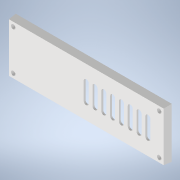
# Autodesk Inventor part: A-04
Saved by Autodesk Inventor 2022.2 (Build 262287000, 287)
## iProperties
Created: 2021-11-25
Part Number: A-04
Material: Generic
Document SubType Name: Modeling
Designer: kfcs7
Density: 1 g/cm^3
Appearance: Default
Author: kfcs7
Autodesk Inventor part; units mm, degrees
ref_plane "YZ Plane" through (0, 0, 0) normal (1, 0, 0) x (0, 1, 0)
ref_plane "XZ Plane" through (0, 0, 0) normal (0, 1, 0) x (-1, 0, 0)
ref_plane "XY Plane" through (0, 0, 0) normal (0, 0, 1) x (1, 0, 0)
sketch "Sketch1" plane through (0, 0, 0) normal (0, 0, 1) x (1, 0, 0)
  circle A0 centre (4, 4) radius 2.25 construction
  line L0 (119, 20) -> (119, 10.0711) construction
  line L1 (119, 10.0711) -> (113.9289, 5) construction
  line L2 (113.9289, 5) -> (10.0711, 5) construction
  line L3 (10.0711, 5) -> (5, 10.0711) construction
  line L4 (5, 10.0711) -> (5, 20) construction
  line L5 (0, 20) -> (5, 20) construction
  line L6 (0, 0) -> (0, 20) construction
  line L7 (124, 0) -> (0, 0) construction
  line L8 (124, 0) -> (124, 20) construction
  line L9 (119, 20) -> (124, 20) construction
  circle A1 centre (120, 4) radius 2.25 construction
  circle A2 centre (120, 36) radius 2.25 construction
  line L10 (119, 29.9289) -> (119, 20) construction
  line L11 (124, 20) -> (119, 20) construction
  line L12 (124, 40) -> (124, 20) construction
  line L13 (0, 40) -> (124, 40) construction
  line L14 (0, 20) -> (0, 40) construction
  line L15 (5, 20) -> (0, 20) construction
  line L16 (5, 20) -> (5, 29.9289) construction
  line L17 (5, 29.9289) -> (10.0711, 35) construction
  line L18 (10.0711, 35) -> (113.9289, 35) construction
  line L19 (113.9289, 35) -> (119, 29.9289) construction
  circle A3 centre (4, 36) radius 2.25 construction
  line L20 (124, 0) -> (0, 0)
  line L21 (0, 0) -> (0, 40)
  line L22 (0, 40) -> (124, 40)
  line L23 (124, 40) -> (124, 0)
  constraints: 8 end point, 2 parallel, 1 horizontal, 1 perpendicular
extrude "Extrusion1" add sketch "Sketch1" along normal blind 6 draft -5
sketch "Sketch4" plane through (0, 0, 0) normal (0, 0, -1) x (-1, 0, 0)
  line L0 (-124, 40) -> (0, 40) construction
  line L1 (-124, 0) -> (-124, 40) construction
  line L2 (0, 0) -> (-124, 0) construction
  line L3 (0, 40) -> (0, 0) construction
  circle A0 centre (-120, 4) radius 2.25 construction
  line L4 (-119, 10.0711) -> (-119, 20) projected
  line L5 (-124, 20) -> (-119, 20) construction
  line L6 (-124, 0) -> (-124, 20) construction
  line L7 (0, 0) -> (-124, 0) construction
  line L8 (0, 20) -> (0, 0) construction
  line L9 (-5, 20) -> (0, 20) construction
  line L10 (-5, 20) -> (-5, 10.0711) projected
  line L11 (-5, 10.0711) -> (-10.0711, 5) projected
  line L12 (-10.0711, 5) -> (-113.9289, 5) projected
  line L13 (-113.9289, 5) -> (-119, 10.0711) projected
  circle A1 centre (-4, 4) radius 2.25 construction
  circle A2 centre (-4, 36) radius 2.25 construction
  line L14 (-119, 20) -> (-119, 29.9289) projected
  line L15 (-119, 29.9289) -> (-113.9289, 35) projected
  line L16 (-113.9289, 35) -> (-10.0711, 35) projected
  line L17 (-10.0711, 35) -> (-5, 29.9289) projected
  line L18 (-5, 29.9289) -> (-5, 20) projected
  line L19 (0, 20) -> (-5, 20) construction
  line L20 (0, 40) -> (0, 20) construction
  line L21 (-124, 40) -> (0, 40) construction
  line L22 (-124, 40) -> (-124, 20) construction
  line L23 (-119, 20) -> (-124, 20) construction
  circle A3 centre (-120, 36) radius 2.25 construction
extrude "Extrusion4" cut sketch "Sketch4" against normal blind 4.5 draft -25
sketch "Sketch5" plane through (0, 0, 6) normal (0, 0, 1) x (1, 0, 0)
  circle A0 centre (120, 4) radius 1.7718 projected
  circle A1 centre (120, 36) radius 1.7718 projected
  circle A2 centre (4, 36) radius 1.7718 projected
  circle A3 centre (4, 4) radius 1.7718 projected
  point P0 (0, 0)
extrude "Extrusion5" cut sketch "Sketch5" against normal through all
sketch "Sketch6" plane through (0, 0, 6) normal (0, 0, 1) x (1, 0, 0)
  circle A0 centre (120, 4) radius 1.7718 projected
  circle A1 centre (4, 36) radius 1.7718 projected
  circle A2 centre (120, 36) radius 1.7718 projected
  circle A3 centre (4, 4) radius 1.7718 projected
  line L0 (123.4751, 39.4751) -> (123.4751, 0.5249) projected
  line L1 (0.5249, 39.4751) -> (123.4751, 39.4751) projected
  line L2 (0.5249, 0.5249) -> (0.5249, 39.4751) projected
  line L3 (123.4751, 0.5249) -> (0.5249, 0.5249) projected
  line L4 (62, 13) -> (62, 27) construction
  line L5 (64, 13) -> (64, 27)
  line L6 (60, 27) -> (60, 13)
  arc A4 (60, 13) -> (64, 13) centre (62, 13) ccw
  arc A5 (64, 27) -> (60, 27) centre (62, 27) ccw
  point P0 (0, 0)
  point P1 (62, 20)
  dimension "d28" = 7
  dimension "d29" = 4
  constraints: 8 end point, 4 point on circle, 4 tangent, 2 centre point, 1 midpoint, 1 parallel, 1 vertical
  measures "d28" distance of point (62, 20) L4.end
  measures "d29" diameter of A5
extrude "Extrusion6" cut sketch "Sketch6" against normal through all contours A4 L6 A5 L5
pattern_linear "Rectangular Pattern1" count 8 spacing 7 along (1, 0, 0) of "Extrusion6"
body "Solid1"
